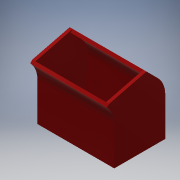
# Autodesk Inventor part: shroud 01 volcano
Saved by Autodesk Inventor 2018.2 (Build 222227000, 227)
## iProperties
Created: 2018-03-01
Part Number: shroud 01 volcano
Material: ABS-Kunststoff
Document SubType Name: Modeling
Designer: Till
Density: 1.06 g/cm^3
Appearance: Rot
Author: Till
Autodesk Inventor part; units mm, degrees
ref_plane "YZ Plane" through (0, 0, 0) normal (1, 0, 0) x (0, 1, 0)
ref_plane "XZ Plane" through (0, 0, 0) normal (0, 1, 0) x (-1, 0, 0)
ref_plane "XY Plane" through (0, 0, 0) normal (0, 0, 1) x (1, 0, 0)
sketch "Skizze1" plane through (0, 0, 0) normal (0, 0, 1) x (1, 0, 0)
  line L0 (-1.2, -1.2) -> (-1.2, -18.6)
  line L1 (-1.2, -18.6) -> (-28.6, -18.6)
  line L2 (-28.6, -18.6) -> (-28.6, -2.2)
  line L3 (0, 0) -> (0, -19.8)
  line L4 (0, -19.8) -> (-29.8, -19.8)
  line L5 (-29.8, -19.8) -> (-29.8, -3.4)
  line L6 (-29.8, -3.4) -> (-35.8, -3.4)
  line L7 (-35.8, -3.4) -> (-35.8, -2.2)
  line L8 (-35.8, -2.2) -> (-28.6, -2.2)
  line L9 (-1.2, -1.2) -> (-35.8, -1.2)
  line L10 (-35.8, -1.2) -> (-35.8, 0)
  line L11 (-35.8, 0) -> (0, 0)
  line L12 (0, -23.76) -> (0, 3.96) projected
  line L13 (-42.96, 0) -> (7.16, 0) projected
  point P0 (7.16, 0)
  dimension "d6" = 17.4
  dimension "d7" = 27.4
  dimension "d8" = 16.4
  dimension "d9" = 90
  dimension "d10" = 6
  dimension "d11" = 90
  dimension "d12" = 1.2
  dimension "d13" = 1.2
  dimension "d14" = 1.2
  dimension "d15" = 1.2
  dimension "d16" = 0
  dimension "d17" = 0
  dimension "d18" = 1.2
  constraints: 24 end point, 8 perpendicular, 2 point on line, 2 vertical, 1 parallel, 1 other
  measures "d6" distance of L0.start L0.end
  measures "d7" distance of L0.end L1.end
  measures "d8" distance of L1.end L2.end
  measures "d9" angle of L1 L2
  measures "d10" distance of L5.end L6.end
  measures "d11" angle of L6 L5
  measures "d12" distance between parallel lines of L1 L4
  measures "d13" distance between parallel lines of L3 L0
  measures "d14" distance between parallel lines of L11 L9
  measures "d15" distance between parallel lines of L2 L5
  measures "d16" distance between parallel lines of L12 L3
  measures "d17" vertical extent of L11
  measures "d18" distance between parallel lines of L8 L6
extrude "Extrusion1" add sketch "Skizze1" along normal blind 9
sketch "Skizze2" plane through (-35.8, -3.4, 0) normal (0, -1, 0) x (1, 0, 0)
  circle A0 centre (3, 3) radius 1.6
  line L0 (0, 9) -> (6, 9) projected
  line L1 (0, 0) -> (0, 9) projected
  line L2 (0, 0) -> (6, 0) projected
  line L3 (6, 9) -> (0, 9)
  line L4 (0, 9) -> (0, 6)
  line L5 (0, 6) -> (6, 6)
  line L6 (6, 6) -> (6, 9)
  point P0 (35.8, 0)
  dimension "d21" = 3.2
  dimension "d23" = 3
  dimension "d75" = 3
  dimension "d76" = 6
  dimension "d77" = 3
  constraints: 8 end point, 2 parallel, 1 centre point, 1 horizontal, 1 perpendicular
  measures "d21" diameter of A0
  measures "d23" distance from line of A0.centre L1
  measures "d75" distance from line of L2 A0.centre
  measures "d76" distance of L5.end L4.end
  measures "d77" distance of L4.end L3.end
extrude "Extrusion2" cut sketch "Skizze2" against normal through all
sketch "Skizze15" plane through (-29.8, -19.8, 0) normal (-1, 0, 0) x (0, 0, 1)
  line L0 (9, 17.6) -> (9, 0) projected
  line L1 (9, 0) -> (19, 0)
  line L2 (9, 0) -> (19, 0) construction
  line L3 (19, 0) -> (21.8284, -2.8284)
  line L4 (21.8284, -2.8284) -> (22.677, -1.9799)
  line L5 (9, 1.2) -> (19.4971, 1.2)
  line L6 (19.4971, 1.2) -> (22.677, -1.9799)
  line L7 (6, 19.8) -> (9, 19.8) projected
  line L8 (9, 19.8) -> (9, 18.6) projected
  line L9 (9, 19.8) -> (9, 18.6)
  line L10 (9, 19.8) -> (19, 19.8)
  line L11 (9, 19.8) -> (19, 19.8) construction
  line L12 (19, 19.8) -> (26.3, 12.5)
  line L13 (9, 18.6) -> (6, 18.6) projected
  line L14 (9, 18.6) -> (18.5029, 18.6)
  line L15 (18.5029, 18.6) -> (25.4515, 11.6515)
  line L16 (25.4515, 11.6515) -> (26.3, 12.5)
  line L17 (28.3, -13.6) -> (28.3, -12.6) projected
  point P0 (0, 19.8)
  dimension "d78" = 10
  dimension "d79" = 0
  dimension "d80" = 4
  dimension "d81" = 135
  dimension "d82" = 1.2
  dimension "d83" = 0
  dimension "d84" = 10
  dimension "d85" = 0
  dimension "d86" = 135
  dimension "d87" = 2
  dimension "d88" = 1.2
  constraints: 26 end point, 6 horizontal, 3 perpendicular, 2 collinear, 1 parallel, 1 point on line, 1 vertical
  measures "d78" distance of L0.end L1.end
  measures "d79" distance between parallel lines of L1 L2
  measures "d80" distance of L1.end L3.end
  measures "d81" angle of L1 L3
  measures "d82" distance of L3.end L4.end
  measures "d83" distance from line of L5 point (9, 1.2)
  measures "d84" distance of L7.end L10.end
  measures "d85" distance between parallel lines of L10 L11
  measures "d86" angle of L10 L12
  measures "d87" distance from line of L17 L12.end
  measures "d88" distance between parallel lines of L12 L15
extrude "Extrusion8" add sketch "Skizze15" against normal up to surface (29.8 mm away)
sketch "Skizze16" plane through (0, -19.8, 0) normal (1, 0, 0) x (0, 0, -1)
  line L0 (-22.677, -1.9799) -> (-19.4971, 1.2) projected
  line L1 (-19.4971, 1.2) -> (-9, 1.2) projected
  line L2 (-9, 1.2) -> (-9, 18.6) projected
  line L3 (-9, 18.6) -> (-18.5029, 18.6) projected
  line L4 (-18.5029, 18.6) -> (-25.4515, 11.6515) projected
  line L5 (-25.4515, 11.6515) -> (-26.3, 12.5) projected
  line L6 (-25.4515, 11.6515) -> (-26.3, 12.5) projected
  line L7 (-22.677, -1.9799) -> (-26.3, 12.5)
  point P0 (0, 19.8)
  constraints: 2 end point
extrude "Extrusion9" add sketch "Skizze16" against normal up to surface (1.2 mm away)
sketch "Skizze17" plane through (-29.8, -19.8, 0) normal (-1, 0, 0) x (0, 0, 1)
  line L0 (9, 17.6) -> (9, 1.2) projected
  line L1 (9, 1.2) -> (19.4971, 1.2) projected
  line L2 (19.4971, 1.2) -> (22.677, -1.9799) projected
  line L3 (25.4515, 11.6515) -> (26.3, 12.5) projected
  line L4 (18.5029, 18.6) -> (25.4515, 11.6515) projected
  line L5 (18.5029, 18.6) -> (6, 18.6) projected
  line L6 (9, 17.6) -> (9, 18.6)
  line L7 (22.677, -1.9799) -> (26.3, 12.5)
  point P0 (0, 19.8)
  constraints: 4 end point, 1 perpendicular, 1 point on line
extrude "Extrusion10" add sketch "Skizze17" against normal up to surface (1.2 mm away)
fillet "Rundung1" radius 10 4 edges at (-14.9, -19.8, 19) (-14.9, 0, 19) (-14.9, -18.6, 19.4971) (-14.9, -1.2, 18.5029)
